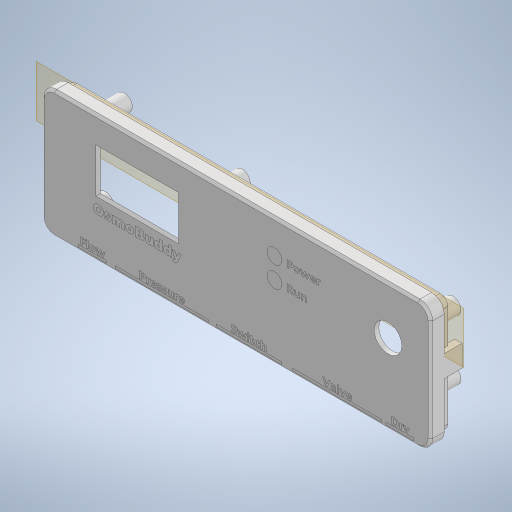
# Autodesk Inventor part: osmobuddy_top
Saved by Autodesk Inventor 2024.3 (Build 283343000, 343)
## iProperties
Created: 2024-10-17
Part Number: osmobuddy_top
Material: Generic
Document SubType Name: Modeling
Designer: atrus
Density: 1 g/cm^3
Appearance: Default
Author: atrus
Autodesk Inventor part; units mm, degrees
(part 1 of 2)
ref_plane "YZ Plane" through (0, 0, 0) normal (1, 0, 0) x (0, 1, 0)
ref_plane "XZ Plane" through (0, 0, 0) normal (0, 1, 0) x (-1, 0, 0)
ref_plane "Work Plane1" through (0, 0, 0) normal (0, 0, 1) x (1, 0, 0)
sketch "Sketch1" plane through (0, 0, 0) normal (0, 0, 1) x (1, 0, 0)
  line L0 (-78.5, 27.45) -> (78.5, 27.45)
  arc A0 (-78.5, 27.45) -> (-83.95, 22) centre (-78.5, 22) ccw
  line L1 (-83.95, -22) -> (-83.95, -15.775)
  arc A1 (-83.95, -22) -> (-78.5, -27.45) centre (-78.5, -22) ccw
  arc A2 (78.5, -27.45) -> (83.95, -22) centre (78.5, -22) ccw
  line L2 (83.95, -3.086) -> (83.95, -22)
  arc A3 (83.95, 22) -> (78.5, 27.45) centre (78.5, 22) ccw
  line L3 (83.95, 22) -> (83.95, -3.086)
  line L4 (-83.95, 22) -> (-83.95, -15.775)
  line L5 (-78.5, -27.45) -> (78.5, -27.45)
  point P0 (0, 0)
extrude "Extrusion1" add sketch "Sketch1" along normal blind 6
sketch "Sketch2" plane through (0, 0, 0) normal (0, 0, -1) x (-1, 0, 0)
  arc A0 (-78.5, 25.5) -> (-82, 22) centre (-78.5, 22) ccw projected
  line L0 (-78.5, 25.5) -> (61.235, 25.5) projected
  arc A1 (82, 22) -> (78.5, 25.5) centre (78.5, 22) ccw projected
  arc A2 (78.5, -25.5) -> (82, -22) centre (78.5, -22) ccw projected
  arc A3 (-82, -22) -> (-78.5, -25.5) centre (-78.5, -22) ccw projected
  line L1 (-82, 22) -> (-82, -22)
  line L2 (-78.5, 25.5) -> (78.5, 25.5)
  line L3 (82, 22) -> (82, -22)
  line L4 (83.95, 22) -> (83.95, -22) projected
  line L5 (78.5, -25.5) -> (-78.5, -25.5)
  line L6 (78.5, -27.45) -> (-78.5, -27.45) projected
  arc A4 (-78.5, 25.3) -> (-81.8, 22) centre (-78.5, 22) ccw
  line L7 (-78.5, 25.3) -> (78.5, 25.3)
  arc A5 (81.8, 22) -> (78.5, 25.3) centre (78.5, 22) ccw
  line L8 (81.8, 22) -> (81.8, -22)
  arc A6 (78.5, -25.3) -> (81.8, -22) centre (78.5, -22) ccw
  line L9 (78.5, -25.3) -> (-78.5, -25.3)
  arc A7 (-81.8, -22) -> (-78.5, -25.3) centre (-78.5, -22) ccw
  line L10 (-81.8, -22) -> (-81.8, 22)
  line L11 (78.5, 24.3) -> (-78.5, 24.3)
  arc A8 (-78.5, 24.3) -> (-80.8, 22) centre (-78.5, 22) ccw
  line L12 (-80.8, 22) -> (-80.8, -22)
  arc A9 (-80.8, -22) -> (-78.5, -24.3) centre (-78.5, -22) ccw
  line L13 (-78.5, -24.3) -> (78.5, -24.3)
  arc A10 (78.5, -24.3) -> (80.8, -22) centre (78.5, -22) ccw
  line L14 (80.8, -22) -> (80.8, 22)
  arc A11 (80.8, 22) -> (78.5, 24.3) centre (78.5, 22) ccw
  point P0 (0, 0)
  dimension "d2" = 0.2
  dimension "d3" = 1
  constraints: 24 end point, 16 point on circle, 8 centre point, 2 parallel, 1 collinear, 14 other
  measures "d2" distance between parallel lines of L0 L7
  measures "d3" distance between parallel lines of L7 L11
extrude "Extrusion2" add sketch "Sketch2" along normal blind 3.7 contours L7 A5 L8 A6 L9 A7 L10 A4
sketch "Sketch12" plane through (0, 0, 0) normal (0, 0, -1) x (-1, 0, 0)
  line L0 (78.5, 24.3) -> (-78.5, 24.3) projected
  arc A0 (-78.5, 24.3) -> (-80.8, 22) centre (-78.5, 22) ccw projected
  line L1 (-80.8, 22) -> (-80.8, -22) projected
  arc A1 (-80.8, -22) -> (-78.5, -24.3) centre (-78.5, -22) ccw projected
  line L2 (-78.5, -24.3) -> (78.5, -24.3) projected
  arc A2 (78.5, -24.3) -> (80.8, -22) centre (78.5, -22) ccw projected
  line L3 (80.8, -22) -> (80.8, 22) projected
  arc A3 (80.8, 22) -> (78.5, 24.3) centre (78.5, 22) ccw projected
  point P0 (0, 0)
extrude "Extrusion12" cut sketch "Sketch12" against normal blind 4
sketch "Sketch3" plane through (0, 0, 4) normal (0, 0, -1) x (-1, 0, 0)
  circle A0 centre (-76.5, 16) radius 1.8 construction
  circle A1 centre (-76.5, -10) radius 1.8 construction
  circle A2 centre (14.5, 18) radius 1.8 construction
  circle A3 centre (14.5, -8) radius 1.8 construction
  circle A4 centre (65.5, 21) radius 1.8 construction
  circle A5 centre (73.5, -20) radius 1.8 construction
  circle A6 centre (-76.5, 16) radius 3.5
  circle A7 centre (-76.5, -10) radius 3.5
  circle A8 centre (14.5, 18) radius 3.5
  circle A9 centre (14.5, -8) radius 3.5
  circle A10 centre (65.5, 21) radius 3.5
  circle A11 centre (73.5, -20) radius 3.5
  point P0 (0, 0)
  dimension "d6" = 7
  constraints: 6 centre point, 6 coincident, 5 equal radius
  measures "d6" diameter of A6
ref_plane "Work Plane2" through (-89.65, -27.5, -11.2032) normal (0, 0, 1) x (1, 0, 0)
extrude "Extrusion3" add sketch "Sketch3" along normal up to surface (15.2032 mm away)
sketch "Sketch4" plane through (0, 0, 6) normal (0, 0, 1) x (1, 0, 0)
  arc A0 (63.3499, 8.5) -> (67.9502, 8.5) centre (65.65, 7) ccw construction
  circle A1 centre (65.65, 7) radius 6
  line L0 (-59.595, 15.12) -> (-25.945, 15.12)
  line L1 (-25.945, 15.12) -> (-25.945, -2.08)
  line L2 (-25.945, -2.08) -> (-59.595, -2.08)
  line L3 (-59.595, -2.08) -> (-59.595, 15.12)
  line L4 (78.5, 27.45) -> (-78.5, 27.45) projected
  circle A2 centre (-44.04, 20) radius 0.508 projected
  circle A3 centre (-41.5, 20) radius 0.508 projected
  line L5 (-44.04, 20) -> (-41.5, 20) construction
  line L6 (-42.77, 20) -> (-42.77, -6.787) construction
  point P0 (0, 0)
  point P1 (-42.77, 15.12)
  dimension "d9" = 12
  dimension "d10" = 12.33
  dimension "d11" = 33.65
  dimension "d12" = 17.2
  constraints: 12 end point, 2 horizontal, 2 midpoint, 2 parallel, 1 centre point, 1 coincident, 1 perpendicular, 1 point on line, 1 vertical
  measures "d9" diameter of A1
  measures "d10" distance from line of L4 L0.end
  measures "d11" distance of L0.start L0.end
  measures "d12" distance of L0.end L1.end
extrude "Extrusion4" cut sketch "Sketch4" against normal blind 10 contours A1 | L0 L1 L2 L3
sketch "Sketch5" plane through (-83.95, -22, 0) normal (-1, 0, 0) x (0, 0, 1)
  line L0 (0, 39.12) -> (0, 20.92) projected
  line L1 (0, 33.7998) -> (-21.3034, 33.7998)
  line L2 (-21.3034, 33.7998) -> (-21.3034, 43.1998)
  line L3 (-21.3034, 43.1998) -> (0, 43.1998)
  line L4 (0, 43.1998) -> (0, 33.7998)
  line L5 (-11.4032, 43.1998) -> (0, 43.1998) construction
  line L6 (-11.2032, 33.9998) -> (-0.2032, 33.9998) construction
  line L7 (-0.2032, 33.9998) -> (-0.2032, 42.9998) projected
  line L8 (-0.2032, 38.4998) -> (5.1502, 38.4998) construction
  line L9 (-3.3332, 27.4) -> (-1.945, 27.4) construction
  line L10 (-1.945, 26.1) -> (-3.3332, 26.1) construction
  line L11 (-3.3332, 27.4) -> (-1.945, 27.4) construction
  line L12 (-1.945, 26.1) -> (-3.3332, 26.1) construction
  line L13 (0, 28.25) -> (-5.2744, 28.25)
  line L14 (-5.2744, 28.25) -> (-5.2744, 25.25)
  line L15 (-5.2744, 25.25) -> (0, 25.25)
  line L16 (0, 25.25) -> (0, 28.25)
  line L17 (-2.6391, 27.4) -> (-2.6391, 26.1) construction
  line L18 (-2.6391, 26.75) -> (7.1194, 26.75) construction
  line L19 (-3.3332, 13.65) -> (-1.945, 13.65) construction
  line L20 (-3.3332, 13.65) -> (-3.3332, 12.35) construction
  line L21 (-1.945, 12.35) -> (-3.3332, 12.35) construction
  line L22 (-1.945, 13.65) -> (-1.945, 12.35) construction
  line L23 (-1.945, 13) -> (5.1502, 13) construction
  line L24 (0, 0) -> (0, 44) projected
  line L25 (0, 14.5) -> (-4.6884, 14.5)
  line L26 (-4.6884, 14.5) -> (-4.6884, 11.5)
  line L27 (-4.6884, 11.5) -> (0, 11.5)
  line L28 (0, 11.5) -> (0, 14.5)
  point P0 (0, 22)
  point P1 (0, 38.4998)
  point P2 (0, 26.75)
  point P3 (-2.6372, 28.25)
  point P4 (0, 13)
  point P5 (-2.3442, 11.5)
  point P6 (-2.3442, 14.5)
  point P7 (0, 11.5)
  dimension "d15" = 3
  dimension "d16" = 3
  constraints: 32 end point, 11 midpoint, 6 horizontal, 6 parallel, 6 point on line, 3 perpendicular, 2 other
  measures "d15" distance from line of L15 point (-2.637, 28.25)
  measures "d16" distance of point (-2.344, 11.5) point (-2.344, 14.5)
extrude "Extrusion5" cut sketch "Sketch5" against normal blind 10
sketch "Sketch6" plane through (0, 0, 0) normal (0, 0, -1) x (-1, 0, 0)
  line L0 (-83.95, -22) -> (-83.95, 22) projected
  line L1 (-83.95, 7.254) -> (-80.8, 7.254)
  line L2 (-80.8, 7.254) -> (-80.8, -2.086)
  line L3 (-80.8, -2.086) -> (-83.95, -2.086)
  line L4 (-83.95, -2.086) -> (-83.95, 7.254)
  line L5 (-80.8, -22) -> (-80.8, 22) projected
  point P0 (0, 0)
  point P1 (-82.95, -2.086)
  point P2 (-82.95, 7.254)
  point P3 (-80.8, 2.584)
  constraints: 8 end point, 4 point on line, 2 parallel, 1 horizontal, 1 midpoint, 1 perpendicular, 2 other
extrude "Extrusion6" add sketch "Sketch6" along normal blind 7.7
sketch "Sketch7" plane through (0, 0, 0) normal (0, 0, -1) x (-1, 0, 0)
  line L0 (78.5, -27.45) -> (-78.5, -27.45) projected
  line L1 (78.5, -24.3) -> (-78.5, -24.3) projected
  line L2 (-65.1727, -27.45) -> (-76.779, -27.45)
  line L3 (-76.779, -27.45) -> (-76.779, -24.3)
  line L4 (-76.779, -24.3) -> (-65.1727, -24.3)
  line L5 (-65.1727, -24.3) -> (-65.1727, -27.45)
  line L6 (-62.93, -27.45) -> (-54.52, -27.45)
  line L7 (-54.52, -27.45) -> (-54.52, -24.3)
  line L8 (-54.52, -24.3) -> (-62.93, -24.3)
  line L9 (-62.93, -24.3) -> (-62.93, -27.45)
  line L10 (-52.5337, -27.45) -> (-44.52, -27.45)
  line L11 (-44.52, -27.45) -> (-44.52, -24.3)
  line L12 (-44.52, -24.3) -> (-52.5337, -24.3)
  line L13 (-52.5337, -24.3) -> (-52.5337, -27.45)
  line L14 (-42.93, -27.45) -> (-34.52, -27.45)
  line L15 (-34.52, -27.45) -> (-34.52, -24.3)
  line L16 (-34.52, -24.3) -> (-42.93, -24.3)
  line L17 (-42.93, -24.3) -> (-42.93, -27.45)
  line L18 (-32.93, -27.45) -> (-24.52, -27.45)
  line L19 (-24.52, -27.45) -> (-24.52, -24.3)
  line L20 (-24.52, -24.3) -> (-32.93, -24.3)
  line L21 (-32.93, -24.3) -> (-32.93, -27.45)
  line L22 (-24.12, -27.45) -> (-20.14, -27.45)
  line L23 (-20.14, -27.45) -> (-20.14, -24.3)
  line L24 (-20.14, -24.3) -> (-24.12, -24.3)
  line L25 (-24.12, -24.3) -> (-24.12, -27.45)
  line L26 (-19.6962, -27.45) -> (-11.33, -27.45)
  line L27 (-11.33, -27.45) -> (-11.33, -24.3)
  line L28 (-11.33, -24.3) -> (-19.6962, -24.3)
  line L29 (-19.6962, -24.3) -> (-19.6962, -27.45)
  line L30 (-9.74, -27.45) -> (-1.33, -27.45)
  line L31 (-1.33, -27.45) -> (-1.33, -24.3)
  line L32 (-1.33, -24.3) -> (-9.74, -24.3)
  line L33 (-9.74, -24.3) -> (-9.74, -27.45)
  line L34 (8.67, -24.3) -> (0, -24.3)
  line L35 (12.221, -27.45) -> (24.241, -27.45)
  line L36 (24.241, -27.45) -> (24.241, -24.3)
  line L37 (24.241, -24.3) -> (12.221, -24.3)
  line L38 (12.221, -24.3) -> (12.221, -27.45)
  line L39 (26.221, -27.45) -> (38.241, -27.45)
  line L40 (38.241, -27.45) -> (38.241, -24.3)
  line L41 (38.241, -24.3) -> (26.221, -24.3)
  line L42 (26.221, -24.3) -> (26.221, -27.45)
  line L43 (40.221, -27.45) -> (52.241, -27.45)
  line L44 (52.241, -27.45) -> (52.241, -24.3)
  line L45 (52.241, -24.3) -> (40.221, -24.3)
  line L46 (40.221, -24.3) -> (40.221, -27.45)
  line L47 (56.021, -27.45) -> (68.241, -27.45)
  line L48 (68.241, -27.45) -> (68.241, -24.3)
  line L49 (68.241, -24.3) -> (56.021, -24.3)
  line L50 (56.021, -24.3) -> (56.021, -27.45)
  line L51 (0.2, -27.45) -> (8.67, -27.45)
  line L52 (8.67, -27.45) -> (8.67, -24.3)
  line L53 (8.67, -24.3) -> (0.2, -24.3)
  line L54 (0.2, -24.3) -> (0.2, -27.45)
  point P0 (0, 0)
  point P1 (68.441, -27.45)
  point P2 (55.821, -27.45)
  point P3 (52.441, -27.45)
  point P4 (40.021, -35.16)
  point P5 (38.441, -27.45)
  point P6 (26.021, -35.16)
  point P7 (24.441, -27.45)
  point P8 (12.021, -35.16)
  point P9 (8.87, -27.45)
  point P10 (0, -27.45)
  point P11 (-1.13, -27.45)
  point P12 (-9.94, -27.45)
  point P13 (-11.13, -27.45)
  point P14 (-19.94, -27.45)
  point P15 (-24.32, -27.45)
  point P16 (-33.13, -27.45)
  point P17 (-34.32, -27.45)
  point P18 (-43.13, -27.45)
  point P19 (-44.32, -27.45)
  point P20 (-53.13, -27.45)
  point P21 (-54.32, -27.45)
  point P22 (-63.13, -27.45)
  point P23 (-64.559, -27.45)
  point P24 (-76.979, -35.16)
  point P25 (52.241, -25.875)
  point P26 (56.021, -25.875)
  point P27 (24.241, -25.875)
  point P28 (12.221, -25.875)
  point P29 (0, -27.45)
  point P30 (-19.6962, -25.875)
  point P31 (-20.14, -25.875)
  point P32 (-24.12, -25.875)
  point P33 (56.021, -24.3)
  point P34 (68.241, -24.3)
  point P35 (40.221, -24.3)
  point P36 (52.241, -24.3)
  point P37 (26.221, -24.3)
  point P38 (38.241, -24.3)
  point P39 (12.221, -24.3)
  point P40 (24.241, -24.3)
  point P41 (0.2, -24.3)
  point P42 (8.67, -24.3)
  point P43 (-9.74, -24.3)
  point P44 (-1.33, -27.45)
  point P45 (-1.33, -24.3)
  point P46 (-19.6962, -24.3)
  point P47 (-11.33, -24.3)
  point P48 (-32.93, -24.3)
  point P49 (-24.52, -24.3)
  point P50 (-42.93, -24.3)
  point P51 (-34.52, -27.45)
  point P52 (-34.52, -24.3)
  point P53 (-52.5337, -24.3)
  point P54 (-44.52, -24.3)
  point P55 (-62.93, -24.3)
  point P56 (-54.52, -24.3)
  point P57 (-65.1727, -24.3)
  point P58 (-76.779, -27.45)
  dimension "d21" = 0.2
  dimension "d22" = 0.2
  dimension "d23" = 0.2
  dimension "d24" = 0.2
  dimension "d25" = 0.2
  dimension "d26" = 0.2
  dimension "d27" = 0.2
  dimension "d28" = 0.2
  dimension "d30" = 0.2
  dimension "d31" = 0.2
  dimension "d32" = 0.2
  dimension "d33" = 0.2
  dimension "d34" = 0.2
  dimension "d35" = 1.575
  dimension "d36" = 0.2
  dimension "d37" = 0.2
  dimension "d38" = 0.2
  dimension "d39" = 0.2
  dimension "d40" = 0.2
  dimension "d41" = 0.2
  dimension "d42" = 0.2
  dimension "d43" = 0.2
  dimension "d44" = 0.2
  dimension "d45" = 0.2
  constraints: 106 end point, 26 parallel, 23 point on line, 13 horizontal, 13 perpendicular, 7 midpoint, 30 other
  measures "d21" distance from line of L46 point (40.021, -35.16)
  measures "d22" horizontal distance of point (52.241, -25.875) point (52.441, -27.45)
  measures "d23" horizontal distance of point (56.021, -25.875) point (55.821, -27.45)
  measures "d24" distance from line of point (68.441, -27.45) L48
  measures "d25" distance from line of point (38.441, -27.45) L40
  measures "d26" distance from line of L42 point (26.021, -35.16)
  measures "d27" horizontal distance of point (24.241, -25.875) point (24.441, -27.45)
  measures "d28" horizontal distance of point (12.021, -35.16) point (12.221, -25.875)
  measures "d30" distance from line of L54 point (0, -27.45)
  measures "d31" distance from line of L52 point (8.87, -27.45)
  measures "d32" distance from line of point (-1.13, -27.45) L31
  measures "d33" distance from line of L33 point (-9.94, -27.45)
  measures "d34" distance from line of point (-11.13, -27.45) L27
  measures "d35" vertical distance of point (-19.696, -25.875) point (-19.94, -27.45)
  measures "d36" horizontal distance of point (-20.14, -25.875) point (-19.94, -27.45)
  measures "d37" horizontal distance of point (-24.12, -25.875) point (-24.32, -27.45)
  measures "d38" distance from line of point (-24.32, -27.45) L19
  measures "d39" distance from line of L21 point (-33.13, -27.45)
  measures "d40" distance from line of point (-34.32, -27.45) L15
  measures "d41" distance from line of L3 point (-76.979, -35.16)
  measures "d42" distance from line of L9 point (-63.13, -27.45)
  measures "d43" distance from line of L7 point (-54.32, -27.45)
  measures "d44" distance from line of point (-44.32, -27.45) L11
  measures "d45" distance from line of point (-43.13, -27.45) L17
extrude "Extrusion7" add sketch "Sketch7" along normal blind 3.7 contours L0 L50 L1 L48 | L0 L46 L1 L44 | L0 L42 L1 L40 | L0 L38 L1 L36 | L0 L54 L1 L52 | L0 L33 L1 L31 | L0 L29 L1 L27 | L0 L21 L1 L19 | L0 L17 L1 L15 | L0 L13 L1 L11 | L0 L9 L1 L7 | L0 L3 L1 L5
sketch "Sketch8" plane through (76.5, 16, -11.2032) normal (0, 0, -1) x (-1, 0, 0)
  circle A0 centre (0, 0) radius 3.5 construction
  circle A1 centre (0, -26) radius 3.5 construction
  circle A2 centre (91, -24) radius 3.5 construction
  circle A3 centre (91, 2) radius 3.5 construction
  circle A4 centre (142, 5) radius 3.5 construction
  circle A5 centre (150, -36) radius 3.5 construction
  circle A6 centre (0, 0) radius 2
  circle A7 centre (0, -26) radius 2
  circle A8 centre (91, 2) radius 2
  circle A9 centre (91, -24) radius 2
  circle A10 centre (142, 5) radius 2
  circle A11 centre (150, -36) radius 2
  point P0 (76.5, -16)
  dimension "d48" = 4
  constraints: 6 centre point, 6 coincident, 5 equal radius
  measures "d48" diameter of A6
extrude "Extrusion8" cut sketch "Sketch8" against normal blind 7
chamfer "Chamfer1" distance 1 angle 45 12 edges at (-42.77, 15.12, 6) (-25.945, 6.52, 6) (-42.77, -2.08, 6) (-59.595, 6.52, 6) (-83.95, 0, 6) (-82.3537, -25.8537, 6) (0, -27.45, 6) (82.3537, -25.8537, 6) (83.95, 0, 6) (82.3537, 25.8537, 6) (0, 27.45, 6) (-82.3537, 25.8537, 6)
sketch "Sketch9" plane through (0, 0, 4) normal (0, 0, -1) x (-1, 0, 0)
  arc A0 (-19.1701, 11.4418) -> (-19.1701, 14.7584) centre (-16.6701, 13.1001) ccw projected
  arc A1 (-19.1701, 2.4418) -> (-19.1701, 5.7584) centre (-16.6701, 4.1001) ccw projected
  circle A2 centre (-16.6701, 13.1001) radius 3.2
  circle A3 centre (-16.6701, 4.1001) radius 3.2
  circle A4 centre (-16.6701, 13.1001) radius 4.2
  circle A5 centre (-16.6701, 4.1001) radius 4.2
  point P0 (0, 0)
  dimension "d54" = 0.2
  dimension "d55" = 1
  constraints: 4 centre point, 2 coincident, 2 equal radius
  measures "d54" radial gap between concentric circles of A2 A0
  measures "d55" radial gap between concentric circles of A4 A2
extrude "Extrusion9" add sketch "Sketch9" along normal blind 10
sketch "Sketch10" plane through (16.6701, 13.1001, 0) normal (0, 0, -1) x (-1, 0, 0)
  circle A0 centre (0, 0) radius 3.2 projected
  circle A1 centre (0, -9) radius 3.2 projected
  point P0 (16.6701, -13.1001)
extrude "Extrusion10" cut sketch "Sketch10" against normal blind 5.6
sketch "Sketch11" plane through (0, 0, 6) normal (0, 0, 1) x (1, 0, 0)
  line L0 (-24.945, -3.08) -> (-24.945, 16.12) projected
  line L1 (-60.595, -3.08) -> (-24.945, -3.08) projected
  line L2 (-60.595, 16.12) -> (-60.595, -3.08) projected
  line L3 (-24.945, 16.12) -> (-60.595, 16.12) projected
  circle A0 centre (65.65, 7) radius 6 projected
  line L4 (-82.95, -22) -> (-82.95, 22) projected
  arc A1 (-82.95, -22) -> (-78.5, -26.45) centre (-78.5, -22) ccw projected
  line L5 (78.5, -26.45) -> (-78.5, -26.45) projected
  arc A2 (78.5, -26.45) -> (82.95, -22) centre (78.5, -22) ccw projected
  line L6 (82.95, 22) -> (82.95, -22) projected
  arc A3 (82.95, 22) -> (78.5, 26.45) centre (78.5, 22) ccw projected
  line L7 (-78.5, 26.45) -> (78.5, 26.45) projected
  arc A4 (-78.5, 26.45) -> (-82.95, 22) centre (-78.5, 22) ccw projected
  circle A5 centre (16.6701, 13.1001) radius 3.2 projected
  circle A6 centre (16.6701, 4.1001) radius 3.2 projected
  point P0 (0, 0)
extrude "Extrusion11" cut sketch "Sketch11" against normal blind 0.001 contours A5 | A6
sketch "Sketch13" plane through (0, 0, 4) normal (0, 0, -1) x (-1, 0, 0)
  line L0 (23.945, 21.12) -> (61.595, 21.12)
  line L1 (61.595, 21.12) -> (61.595, -8.08)
  line L2 (61.595, -8.08) -> (23.945, -8.08)
  line L3 (23.945, -8.08) -> (23.945, 21.12)
  line L4 (59.595, -2.08) -> (25.945, -2.08) projected
  line L5 (25.945, -2.08) -> (25.945, 15.12) projected
  line L6 (59.595, 15.12) -> (59.595, -2.08) projected
  line L7 (25.945, 15.12) -> (59.595, 15.12) projected
  point P0 (0, 0)
  point P1 (42.77, -2.08)
  point P2 (42.77, -8.08)
  point P3 (42.77, 15.12)
  dimension "d64" = 6
  dimension "d65" = 2
  dimension "d66" = 2
  dimension "d67" = 6
  constraints: 8 end point, 3 midpoint, 2 parallel, 1 horizontal, 1 perpendicular
  measures "d64" distance of point (42.77, -2.08) point (42.77, -8.08)
  measures "d65" distance between parallel lines of L5 L3
  measures "d66" distance between parallel lines of L6 L1
  measures "d67" distance from line of point (42.77, 15.12) L0
extrude "Extrusion13" cut sketch "Sketch13" against normal blind 1
sketch "Sketch14" plane through (0, 0, 6) normal (0, 0, 1) x (1, 0, 0)
  line L0 (-68.241, -24.56) -> (-56.021, -24.56) construction
  line L1 (-68.241, -28.56) -> (-68.241, -35.16) construction
  line L2 (-56.021, -28.56) -> (-56.021, -35.16) construction
  line L3 (-52.241, -28.56) -> (-52.241, -35.16) construction
  line L4 (-12.021, -28.56) -> (-12.021, -35.16) construction
  line L5 (-8.67, -34.606) -> (-8.67, -28.806) construction
  line L6 (19.74, -34.606) -> (19.74, -28.806) construction
  line L7 (-52.241, -24.56) -> (-12.021, -24.56) construction
  line L8 (-8.67, -24.56) -> (19.74, -24.56) construction
  line L9 (62.93, -34.606) -> (62.93, -28.806) construction
  line L10 (64.759, -28.56) -> (64.759, -35.16) construction
  line L11 (76.979, -28.56) -> (76.979, -35.16) construction
  line L12 (24.52, -24.56) -> (62.93, -24.56) construction
  line L13 (24.52, -34.606) -> (24.52, -28.806) construction
  line L14 (64.759, -28.56) -> (64.759, -35.16) construction
  line L15 (76.979, -28.56) -> (76.979, -35.16) construction
  line L16 (64.759, -24.56) -> (76.979, -24.56) construction
  line L17 (-52.241, -24.96) -> (-12.021, -24.96)
  line L18 (-12.021, -24.96) -> (-12.021, -25.96)
  line L19 (-12.021, -25.96) -> (-52.241, -25.96)
  line L20 (-52.241, -25.96) -> (-52.241, -24.96)
  line L21 (-68.241, -25.3) -> (-68.241, -27.45) projected
  line L22 (-56.021, -24.96) -> (-68.241, -24.96)
  line L23 (-68.241, -24.96) -> (-68.241, -25.96)
  line L24 (-68.241, -25.96) -> (-56.021, -25.96)
  line L25 (-56.021, -25.96) -> (-56.021, -24.96)
  line L26 (-8.67, -25.3) -> (-8.67, -27.45) projected
  line L27 (-8.67, -25.96) -> (19.74, -25.96)
  line L28 (19.74, -25.96) -> (19.74, -24.96)
  line L29 (19.74, -24.96) -> (-8.67, -24.96)
  line L30 (-8.67, -24.96) -> (-8.67, -25.96)
  line L31 (24.52, -25.96) -> (62.93, -25.96)
  line L32 (62.93, -25.96) -> (62.93, -24.96)
  line L33 (62.93, -24.96) -> (24.52, -24.96)
  line L34 (24.52, -24.96) -> (24.52, -25.96)
  line L35 (76.779, -25.3) -> (76.779, -27.45) projected
  line L36 (64.759, -24.96) -> (76.779, -24.96)
  line L37 (76.779, -24.96) -> (76.779, -25.96)
  line L38 (76.779, -25.96) -> (64.759, -25.96)
  line L39 (64.759, -25.96) -> (64.759, -24.96)
  circle A0 centre (16.6701, 13.1001) radius 3.2 construction
  circle A1 centre (16.6701, 4.1001) radius 3.2 construction
  line L40 (16.6701, 13.1001) -> (16.6701, 9.9001) construction
  line L41 (16.6701, 4.1001) -> (16.6701, 0.9001) construction
  line L42 (16.6701, 2.5001) -> (21.6701, 2.5001) construction
  line L43 (16.6701, 11.5001) -> (21.6701, 11.5001) construction
  line L44 (-61.8904, -9.6935) -> (-23.2153, -9.6935) construction
  line L45 (-64.9786, -22.076) -> (-64.9786, -21.51)
  line L46 (-64.9786, -21.51) -> (-67.2837, -21.51)
  line L47 (-67.2837, -21.51) -> (-67.2837, -24.56)
  line L48 (-67.2837, -24.56) -> (-66.577, -24.56)
  line L49 (-66.577, -24.56) -> (-66.577, -23.4485)
  line L50 (-66.577, -23.4485) -> (-65.1663, -23.4485)
  line L51 (-65.1663, -23.4485) -> (-65.1663, -22.8825)
  line L52 (-65.1663, -22.8825) -> (-66.577, -22.8825)
  line L53 (-66.577, -22.8825) -> (-66.577, -22.076)
  line L54 (-66.577, -22.076) -> (-64.9786, -22.076)
  line L55 (-64.5475, -24.56) -> (-63.8672, -24.56)
  line L56 (-63.8672, -24.56) -> (-63.8672, -21.3282)
  line L57 (-63.8672, -21.3282) -> (-64.5475, -21.3282)
  line L58 (-64.5475, -21.3282) -> (-64.5475, -24.56)
  spline S0 degree 2 poles (-62.1222, -24.5952) (-61.7468, -24.5923) (-61.1691, -24.2873) (-60.8406, -23.7447) (-60.8377, -23.3869) knots 0 0 0 1 2 3 3 3
  spline S1 degree 2 poles (-60.8377, -23.3869) (-60.8406, -23.0321) (-61.1691, -22.4895) (-61.7468, -22.1845) (-62.1222, -22.1816) knots 0 0 0 1 2 3 3 3
  spline S2 degree 2 poles (-62.1222, -22.1816) (-62.4976, -22.1845) (-63.0783, -22.4895) (-63.4097, -23.0321) (-63.4126, -23.3869) knots 0 0 0 1 2 3 3 3
  spline S3 degree 2 poles (-63.4126, -23.3869) (-63.4097, -23.7447) (-63.0783, -24.2873) (-62.4976, -24.5923) (-62.1222, -24.5952) knots 0 0 0 1 2 3 3 3
  spline S4 degree 2 poles (-62.1222, -24.038) (-62.3832, -24.035) (-62.7175, -23.6949) (-62.7234, -23.3869) knots 0 0 0 1 2 2 2
  spline S5 degree 2 poles (-62.7234, -23.3869) (-62.7175, -23.0819) (-62.3832, -22.7417) (-62.1222, -22.7388) knots 0 0 0 1 2 2 2
  spline S6 degree 2 poles (-62.1222, -22.7388) (-61.8641, -22.7417) (-61.5327, -23.0819) (-61.5269, -23.3869) knots 0 0 0 1 2 2 2
  spline S7 degree 2 poles (-61.5269, -23.3869) (-61.5327, -23.6949) (-61.8641, -24.035) (-62.1222, -24.038) knots 0 0 0 1 2 2 2
  line L59 (-57.2217, -22.2168) -> (-57.7935, -23.8034)
  line L60 (-57.7935, -23.8034) -> (-58.3508, -22.2168)
  line L61 (-58.3508, -22.2168) -> (-58.9256, -22.2168)
  line L62 (-58.9256, -22.2168) -> (-59.5004, -23.8034)
  line L63 (-59.5004, -23.8034) -> (-60.0547, -22.2168)
  line L64 (-60.0547, -22.2168) -> (-60.694, -22.2168)
  line L65 (-60.694, -22.2168) -> (-59.8494, -24.56)
  line L66 (-59.8494, -24.56) -> (-59.1954, -24.56)
  line L67 (-59.1954, -24.56) -> (-58.6499, -23.1054)
  line L68 (-58.6499, -23.1054) -> (-58.1249, -24.56)
  line L69 (-58.1249, -24.56) -> (-57.471, -24.56)
  line L70 (-57.471, -24.56) -> (-56.6205, -22.2168)
  line L71 (-56.6205, -22.2168) -> (-57.2217, -22.2168)
  line L72 (-40.4789, -21.51) -> (-41.7986, -21.51)
  line L73 (-41.7986, -21.51) -> (-41.7986, -24.56)
  line L74 (-41.7986, -24.56) -> (-41.0918, -24.56)
  line L75 (-41.0918, -24.56) -> (-41.0918, -23.7183)
  line L76 (-41.0918, -23.7183) -> (-40.4789, -23.7183)
  spline S8 degree 2 poles (-40.4789, -23.7183) (-39.8601, -23.7125) (-39.1592, -23.1318) (-39.1533, -22.6156) knots 0 0 0 1 2 2 2
  spline S9 degree 2 poles (-39.1533, -22.6156) (-39.1592, -22.0995) (-39.8601, -21.5159) (-40.4789, -21.51) knots 0 0 0 1 2 2 2
  line L77 (-40.517, -23.1435) -> (-41.0918, -23.1435)
  line L78 (-41.0918, -23.1435) -> (-41.0918, -22.0848)
  line L79 (-41.0918, -22.0848) -> (-40.517, -22.0848)
  spline S10 degree 2 poles (-40.517, -22.0848) (-40.1944, -22.0877) (-39.8689, -22.3634) (-39.8689, -22.6156) knots 0 0 0 1 2 2 2
  spline S11 degree 2 poles (-39.8689, -22.6156) (-39.8689, -22.8678) (-40.1944, -23.1406) (-40.517, -23.1435) knots 0 0 0 1 2 2 2
  line L80 (-38.0096, -22.5247) -> (-38.0096, -22.2168)
  line L81 (-38.0096, -22.2168) -> (-38.6577, -22.2168)
  line L82 (-38.6577, -22.2168) -> (-38.6577, -24.56)
  line L83 (-38.6577, -24.56) -> (-37.9773, -24.56)
  line L84 (-37.9773, -24.56) -> (-37.9773, -23.4544)
  spline S12 degree 2 poles (-37.9773, -23.4544) (-37.9744, -23.1171) (-37.6401, -22.8004) (-37.3556, -22.8004) knots 0 0 0 1 2 2 2
  spline S13 degree 2 poles (-37.3556, -22.8004) (-37.3175, -22.8004) (-37.2442, -22.8063) (-37.2031, -22.8092) knots 0 0 0 1 2 2 2
  line L85 (-37.2031, -22.8092) -> (-37.2031, -22.1816)
  spline S14 degree 2 poles (-37.2031, -22.1816) (-37.4758, -22.1816) (-37.8835, -22.3546) (-38.0096, -22.5247) knots 0 0 0 1 2 2 2
  spline S15 degree 2 poles (-34.4845, -23.3987) (-34.4874, -23.0174) (-34.8071, -22.4749) (-35.3555, -22.1845) (-35.7045, -22.1816) knots 0 0 0 1 2 3 3 3
  spline S16 degree 2 poles (-35.7045, -22.1816) (-36.0652, -22.1845) (-36.6254, -22.4925) (-36.9509, -23.035) (-36.9538, -23.3899) knots 0 0 0 1 2 3 3 3
  spline S17 degree 2 poles (-36.9538, -23.3899) (-36.9509, -23.7388) (-36.6224, -24.2814) (-36.0242, -24.5923) (-35.6165, -24.5952) knots 0 0 0 1 2 3 3 3
  spline S18 degree 2 poles (-35.6165, -24.5952) (-35.2998, -24.5952) (-34.8129, -24.4016) (-34.6487, -24.2169) knots 0 0 0 1 2 2 2
  line L86 (-34.6487, -24.2169) -> (-35.0124, -23.8239)
  spline S19 degree 2 poles (-35.0124, -23.8239) (-35.1297, -23.9383) (-35.4142, -24.0497) (-35.5989, -24.0497) knots 0 0 0 1 2 2 2
  spline S20 degree 2 poles (-35.5989, -24.0497) (-35.8687, -24.0468) (-36.2177, -23.8004) (-36.2705, -23.5805) knots 0 0 0 1 2 2 2
  line L87 (-36.2705, -23.5805) -> (-34.4992, -23.5805)
  spline S21 degree 2 poles (-34.4992, -23.5805) (-34.4933, -23.5365) (-34.4845, -23.4368) (-34.4845, -23.3987) knots 0 0 0 1 2 2 2
  spline S22 degree 2 poles (-35.6986, -22.6948) (-35.4669, -22.6977) (-35.1649, -22.9588) (-35.1238, -23.1846) knots 0 0 0 1 2 2 2
  line L88 (-35.1238, -23.1846) -> (-36.2793, -23.1846)
  spline S23 degree 2 poles (-36.2793, -23.1846) (-36.2412, -22.9558) (-35.9332, -22.6977) (-35.6986, -22.6948) knots 0 0 0 1 2 2 2
  spline S24 degree 2 poles (-33.244, -24.5952) (-32.7161, -24.5893) (-32.1413, -24.1846) (-32.1383, -23.8503) knots 0 0 0 1 2 2 2
  spline S25 degree 2 poles (-32.1383, -23.8503) (-32.1442, -23.5775) (-32.4287, -23.296) (-32.848, -23.1787) (-33.2674, -23.123) (-33.549, -23.0291) (-33.5548, -22.9148) knots 0 0 0 1 2 3 4 5 5 5
  spline S26 degree 2 poles (-33.5548, -22.9148) (-33.5578, -22.8209) (-33.3466, -22.6977) (-33.1179, -22.6948) knots 0 0 0 1 2 2 2
  spline S27 degree 2 poles (-33.1179, -22.6948) (-32.9566, -22.6919) (-32.6164, -22.774) (-32.4433, -22.8708) knots 0 0 0 1 2 2 2
  line L89 (-32.4433, -22.8708) -> (-32.2175, -22.3869)
  spline S28 degree 2 poles (-32.2175, -22.3869) (-32.3876, -22.2872) (-32.8715, -22.1816) (-33.1179, -22.1816) knots 0 0 0 1 2 2 2
  spline S29 degree 2 poles (-33.1179, -22.1816) (-33.634, -22.1875) (-34.2, -22.601) (-34.2029, -22.9412) knots 0 0 0 1 2 2 2
  spline S30 degree 2 poles (-34.2029, -22.9412) (-34.1971, -23.2168) (-33.9126, -23.5013) (-33.4932, -23.6215) (-33.0739, -23.6714) (-32.7923, -23.7594) (-32.7865, -23.8679) knots 0 0 0 1 2 3 4 5 5 5
  spline S31 degree 2 poles (-32.7865, -23.8679) (-32.7835, -23.9676) (-32.9859, -24.082) (-33.2176, -24.082) knots 0 0 0 1 2 2 2
  spline S32 degree 2 poles (-33.2176, -24.082) (-33.4404, -24.082) (-33.8716, -23.9588) (-34.0329, -23.8562) knots 0 0 0 1 2 2 2
  line L90 (-34.0329, -23.8562) -> (-34.2587, -24.343)
  spline S33 degree 2 poles (-34.2587, -24.343) (-34.0915, -24.4515) (-33.549, -24.5923) (-33.244, -24.5952) knots 0 0 0 1 2 2 2
  spline S34 degree 2 poles (-30.9301, -24.5952) (-30.4022, -24.5893) (-29.8274, -24.1846) (-29.8244, -23.8503) knots 0 0 0 1 2 2 2
  spline S35 degree 2 poles (-29.8244, -23.8503) (-29.8303, -23.5775) (-30.1148, -23.296) (-30.5342, -23.1787) (-30.9535, -23.123) (-31.2351, -23.0291) (-31.2409, -22.9148) knots 0 0 0 1 2 3 4 5 5 5
  spline S36 degree 2 poles (-31.2409, -22.9148) (-31.2439, -22.8209) (-31.0327, -22.6977) (-30.804, -22.6948) knots 0 0 0 1 2 2 2
  spline S37 degree 2 poles (-30.804, -22.6948) (-30.6427, -22.6919) (-30.3025, -22.774) (-30.1294, -22.8708) knots 0 0 0 1 2 2 2
  line L91 (-30.1294, -22.8708) -> (-29.9036, -22.3869)
  spline S38 degree 2 poles (-29.9036, -22.3869) (-30.0737, -22.2872) (-30.5576, -22.1816) (-30.804, -22.1816) knots 0 0 0 1 2 2 2
  spline S39 degree 2 poles (-30.804, -22.1816) (-31.3201, -22.1875) (-31.8861, -22.601) (-31.8891, -22.9412) knots 0 0 0 1 2 2 2
  spline S40 degree 2 poles (-31.8891, -22.9412) (-31.8832, -23.2168) (-31.5987, -23.5013) (-31.1793, -23.6215) (-30.76, -23.6714) (-30.4784, -23.7594) (-30.4726, -23.8679) knots 0 0 0 1 2 3 4 5 5 5
  spline S41 degree 2 poles (-30.4726, -23.8679) (-30.4696, -23.9676) (-30.672, -24.082) (-30.9037, -24.082) knots 0 0 0 1 2 2 2
  spline S42 degree 2 poles (-30.9037, -24.082) (-31.1266, -24.082) (-31.5577, -23.9588) (-31.719, -23.8562) knots 0 0 0 1 2 2 2
  line L92 (-31.719, -23.8562) -> (-31.9448, -24.343)
  spline S43 degree 2 poles (-31.9448, -24.343) (-31.7776, -24.4515) (-31.2351, -24.5923) (-30.9301, -24.5952) knots 0 0 0 1 2 2 2
  line L93 (-27.7246, -22.2168) -> (-27.7246, -23.3781)
  spline S44 degree 2 poles (-27.7246, -23.3781) (-27.7276, -23.7007) (-28.0238, -24.0087) (-28.2642, -24.0087) knots 0 0 0 1 2 2 2
  spline S45 degree 2 poles (-28.2642, -24.0087) (-28.493, -24.0116) (-28.7393, -23.7359) (-28.7393, -23.4426) knots 0 0 0 1 2 2 2
  line L94 (-28.7393, -23.4426) -> (-28.7393, -22.2168)
  line L95 (-28.7393, -22.2168) -> (-29.4197, -22.2168)
  line L96 (-29.4197, -22.2168) -> (-29.4197, -23.5424)
  spline S46 degree 2 poles (-29.4197, -23.5424) (-29.4168, -23.9031) (-29.1646, -24.3694) (-28.7129, -24.5952) (-28.4167, -24.5952) knots 0 0 0 1 2 3 3 3
  spline S47 degree 2 poles (-28.4167, -24.5952) (-28.1997, -24.5952) (-27.8243, -24.4368) (-27.6894, -24.2814) knots 0 0 0 1 2 2 2
  line L97 (-27.6894, -24.2814) -> (-27.6894, -24.56)
  line L98 (-27.6894, -24.56) -> (-27.0442, -24.56)
  line L99 (-27.0442, -24.56) -> (-27.0442, -22.2168)
  line L100 (-27.0442, -22.2168) -> (-27.7246, -22.2168)
  line L101 (-25.7656, -22.5247) -> (-25.7656, -22.2168)
  line L102 (-25.7656, -22.2168) -> (-26.4137, -22.2168)
  line L103 (-26.4137, -22.2168) -> (-26.4137, -24.56)
  line L104 (-26.4137, -24.56) -> (-25.7333, -24.56)
  line L105 (-25.7333, -24.56) -> (-25.7333, -23.4544)
  spline S48 degree 2 poles (-25.7333, -23.4544) (-25.7304, -23.1171) (-25.3961, -22.8004) (-25.1116, -22.8004) knots 0 0 0 1 2 2 2
  spline S49 degree 2 poles (-25.1116, -22.8004) (-25.0735, -22.8004) (-25.0002, -22.8063) (-24.9591, -22.8092) knots 0 0 0 1 2 2 2
  line L106 (-24.9591, -22.8092) -> (-24.9591, -22.1816)
  spline S50 degree 2 poles (-24.9591, -22.1816) (-25.2318, -22.1816) (-25.6395, -22.3546) (-25.7656, -22.5247) knots 0 0 0 1 2 2 2
  spline S51 degree 2 poles (-22.2405, -23.3987) (-22.2434, -23.0174) (-22.5631, -22.4749) (-23.1115, -22.1845) (-23.4605, -22.1816) knots 0 0 0 1 2 3 3 3
  spline S52 degree 2 poles (-23.4605, -22.1816) (-23.8212, -22.1845) (-24.3814, -22.4925) (-24.7069, -23.035) (-24.7098, -23.3899) knots 0 0 0 1 2 3 3 3
  spline S53 degree 2 poles (-24.7098, -23.3899) (-24.7069, -23.7388) (-24.3784, -24.2814) (-23.7802, -24.5923) (-23.3725, -24.5952) knots 0 0 0 1 2 3 3 3
  spline S54 degree 2 poles (-23.3725, -24.5952) (-23.0558, -24.5952) (-22.569, -24.4016) (-22.4047, -24.2169) knots 0 0 0 1 2 2 2
  line L107 (-22.4047, -24.2169) -> (-22.7684, -23.8239)
  spline S55 degree 2 poles (-22.7684, -23.8239) (-22.8857, -23.9383) (-23.1702, -24.0497) (-23.3549, -24.0497) knots 0 0 0 1 2 2 2
  spline S56 degree 2 poles (-23.3549, -24.0497) (-23.6247, -24.0468) (-23.9737, -23.8004) (-24.0265, -23.5805) knots 0 0 0 1 2 2 2
  line L108 (-24.0265, -23.5805) -> (-22.2552, -23.5805)
  spline S57 degree 2 poles (-22.2552, -23.5805) (-22.2493, -23.5365) (-22.2405, -23.4368) (-22.2405, -23.3987) knots 0 0 0 1 2 2 2
  spline S58 degree 2 poles (-23.4546, -22.6948) (-23.2229, -22.6977) (-22.9209, -22.9588) (-22.8798, -23.1846) knots 0 0 0 1 2 2 2
  line L109 (-22.8798, -23.1846) -> (-24.0353, -23.1846)
  spline S59 degree 2 poles (-24.0353, -23.1846) (-23.9972, -22.9558) (-23.6892, -22.6977) (-23.4546, -22.6948) knots 0 0 0 1 2 2 2
  spline S60 degree 2 poles (-0.9243, -24.6128) (-0.4902, -24.6099) (0.0846, -24.3518) (0.3691, -23.9265) (0.3691, -23.6685) knots 0 0 0 1 2 3 3 3
  spline S61 degree 2 poles (0.3691, -23.6685) (0.3632, -23.3371) (0.0083, -22.9763) (-0.5195, -22.8033) (-1.0445, -22.6948) (-1.3994, -22.5364) (-1.4052, -22.3722) knots 0 0 0 1 2 3 4 5 5 5
  spline S62 degree 2 poles (-1.4052, -22.3722) (-1.4081, -22.2256) (-1.1354, -22.0262) (-0.8245, -22.0232) knots 0 0 0 1 2 2 2
  spline S63 degree 2 poles (-0.8245, -22.0232) (-0.6222, -22.0232) (-0.1911, -22.1435) (0.0201, -22.2637) knots 0 0 0 1 2 2 2
  line L110 (0.0201, -22.2637) -> (0.2371, -21.727)
  spline S64 degree 2 poles (0.2371, -21.727) (0.023, -21.5921) (-0.5283, -21.4572) (-0.8216, -21.4572) knots 0 0 0 1 2 2 2
  spline S65 degree 2 poles (-0.8216, -21.4572) (-1.2527, -21.4601) (-1.8246, -21.7153) (-2.1061, -22.1435) (-2.1061, -22.4074) knots 0 0 0 1 2 3 3 3
  spline S66 degree 2 poles (-2.1061, -22.4074) (-2.1003, -22.7417) (-1.7454, -23.1054) (-1.2175, -23.2843) (-0.6926, -23.3928) (-0.3377, -23.5541) (-0.3319, -23.7213) knots 0 0 0 1 2 3 4 5 5 5
  spline S67 degree 2 poles (-0.3319, -23.7213) (-0.3289, -23.862) (-0.6105, -24.0438) (-0.9213, -24.0468) knots 0 0 0 1 2 2 2
  spline S68 degree 2 poles (-0.9213, -24.0468) (-1.1999, -24.0438) (-1.7307, -23.8708) (-1.9272, -23.73) knots 0 0 0 1 2 2 2
  line L111 (-1.9272, -23.73) -> (-2.1677, -24.2609)
  spline S69 degree 2 poles (-2.1677, -24.2609) (-1.9566, -24.4192) (-1.2967, -24.6099) (-0.9243, -24.6128) knots 0 0 0 1 2 2 2
  line L112 (3.9645, -22.2168) -> (3.3927, -23.8034)
  line L113 (3.3927, -23.8034) -> (2.8355, -22.2168)
  line L114 (2.8355, -22.2168) -> (2.2606, -22.2168)
  line L115 (2.2606, -22.2168) -> (1.6858, -23.8034)
  line L116 (1.6858, -23.8034) -> (1.1316, -22.2168)
  line L117 (1.1316, -22.2168) -> (0.4922, -22.2168)
  line L118 (0.4922, -22.2168) -> (1.3369, -24.56)
  line L119 (1.3369, -24.56) -> (1.9908, -24.56)
  line L120 (1.9908, -24.56) -> (2.5363, -23.1054)
  line L121 (2.5363, -23.1054) -> (3.0613, -24.56)
  line L122 (3.0613, -24.56) -> (3.7153, -24.56)
  line L123 (3.7153, -24.56) -> (4.5657, -22.2168)
  line L124 (4.5657, -22.2168) -> (3.9645, -22.2168)
  line L125 (4.8825, -24.56) -> (5.5629, -24.56)
  line L126 (5.5629, -24.56) -> (5.5629, -22.2168)
  line L127 (5.5629, -22.2168) -> (4.8825, -22.2168)
  line L128 (4.8825, -22.2168) -> (4.8825, -24.56)
  spline S70 degree 2 poles (5.2227, -21.8883) (5.4133, -21.8854) (5.642, -21.6684) (5.645, -21.4983) knots 0 0 0 1 2 2 2
  spline S71 degree 2 poles (5.645, -21.4983) (5.642, -21.337) (5.4133, -21.1346) (5.2227, -21.1317) knots 0 0 0 1 2 2 2
  spline S72 degree 2 poles (5.2227, -21.1317) (5.032, -21.1346) (4.8033, -21.3458) (4.8004, -21.51) knots 0 0 0 1 2 2 2
  spline S73 degree 2 poles (4.8004, -21.51) (4.8033, -21.6742) (5.032, -21.8854) (5.2227, -21.8883) knots 0 0 0 1 2 2 2
  spline S74 degree 2 poles (7.5219, -23.9676) (7.4662, -24.0116) (7.3225, -24.0556) (7.2462, -24.0556) knots 0 0 0 1 2 2 2
  spline S75 degree 2 poles (7.2462, -24.0556) (7.1084, -24.0556) (6.9559, -23.8972) (6.9559, -23.7476) knots 0 0 0 1 2 2 2
  line L129 (6.9559, -23.7476) -> (6.9559, -22.7916)
  line L130 (6.9559, -22.7916) -> (7.5395, -22.7916)
  line L131 (7.5395, -22.7916) -> (7.5395, -22.2696)
  line L132 (7.5395, -22.2696) -> (6.9559, -22.2696)
  line L133 (6.9559, -22.2696) -> (6.9559, -21.7006)
  line L134 (6.9559, -21.7006) -> (6.2755, -21.7006)
  line L135 (6.2755, -21.7006) -> (6.2755, -22.2696)
  line L136 (6.2755, -22.2696) -> (5.9148, -22.2696)
  line L137 (5.9148, -22.2696) -> (5.9148, -22.7916)
  line L138 (5.9148, -22.7916) -> (6.2755, -22.7916)
  line L139 (6.2755, -22.7916) -> (6.2755, -23.7535)
  spline S76 degree 2 poles (6.2755, -23.7535) (6.2784, -24.1729) (6.733, -24.5952) (7.1524, -24.5952) knots 0 0 0 1 2 2 2
  spline S77 degree 2 poles (7.1524, -24.5952) (7.3107, -24.5952) (7.5981, -24.5219) (7.7037, -24.4486) knots 0 0 0 1 2 2 2
  line L140 (7.7037, -24.4486) -> (7.5219, -23.9676)
  spline S78 degree 2 poles (9.2199, -24.5952) (9.5924, -24.5923) (10.1379, -24.2873) (10.2698, -24.0028) knots 0 0 0 1 2 2 2
  line L141 (10.2698, -24.0028) -> (9.7419, -23.7154)
  spline S79 degree 2 poles (9.7419, -23.7154) (9.6452, -23.8855) (9.3754, -24.038) (9.2141, -24.038) knots 0 0 0 1 2 2 2
  spline S80 degree 2 poles (9.2141, -24.038) (8.9501, -24.035) (8.607, -23.6978) (8.6011, -23.3869) knots 0 0 0 1 2 2 2
  spline S81 degree 2 poles (8.6011, -23.3869) (8.607, -23.079) (8.9501, -22.7417) (9.2141, -22.7388) knots 0 0 0 1 2 2 2
  spline S82 degree 2 poles (9.2141, -22.7388) (9.3754, -22.7388) (9.6452, -22.8942) (9.7419, -23.0614) knots 0 0 0 1 2 2 2
  line L142 (9.7419, -23.0614) -> (10.2698, -22.7769)
  spline S83 degree 2 poles (10.2698, -22.7769) (10.1379, -22.4895) (9.5924, -22.1845) (9.2199, -22.1816) knots 0 0 0 1 2 2 2
  spline S84 degree 2 poles (9.2199, -22.1816) (8.8357, -22.1845) (8.2492, -22.4895) (7.9149, -23.0321) (7.9119, -23.3869) knots 0 0 0 1 2 3 3 3
  spline S85 degree 2 poles (7.9119, -23.3869) (7.9149, -23.7447) (8.2492, -24.2873) (8.8357, -24.5923) (9.2199, -24.5952) knots 0 0 0 1 2 3 3 3
  spline S86 degree 2 poles (12.0881, -22.1816) (11.8594, -22.1816) (11.481, -22.3224) (11.3432, -22.4602) knots 0 0 0 1 2 2 2
  line L143 (11.3432, -22.4602) -> (11.3432, -21.3282)
  line L144 (11.3432, -21.3282) -> (10.6628, -21.3282)
  line L145 (10.6628, -21.3282) -> (10.6628, -24.56)
  line L146 (10.6628, -24.56) -> (11.3432, -24.56)
  line L147 (11.3432, -24.56) -> (11.3432, -23.3987)
  spline S87 degree 2 poles (11.3432, -23.3987) (11.3461, -23.0761) (11.6541, -22.7681) (11.9033, -22.7681) knots 0 0 0 1 2 2 2
  spline S88 degree 2 poles (11.9033, -22.7681) (12.1321, -22.7681) (12.3784, -23.0379) (12.3784, -23.3224) knots 0 0 0 1 2 2 2
  line L148 (12.3784, -23.3224) -> (12.3784, -24.56)
  line L149 (12.3784, -24.56) -> (13.0588, -24.56)
  line L150 (13.0588, -24.56) -> (13.0588, -23.2168)
  spline S89 degree 2 poles (13.0588, -23.2168) (13.0559, -22.862) (12.8037, -22.4015) (12.3667, -22.1816) (12.0881, -22.1816) knots 0 0 0 1 2 3 3 3
  line L151 (40.0181, -21.51) -> (39.0767, -23.689)
  line L152 (39.0767, -23.689) -> (38.15, -21.51)
  line L153 (38.15, -21.51) -> (37.3875, -21.51)
  line L154 (37.3875, -21.51) -> (38.7013, -24.56)
  line L155 (38.7013, -24.56) -> (39.3993, -24.56)
  line L156 (39.3993, -24.56) -> (40.719, -21.51)
  line L157 (40.719, -21.51) -> (40.0181, -21.51)
  spline S90 degree 2 poles (42.0182, -22.1816) (41.7337, -22.1816) (41.2058, -22.3282) (41.0093, -22.4631) knots 0 0 0 1 2 2 2
  line L158 (41.0093, -22.4631) -> (41.2527, -22.9412)
  spline S91 degree 2 poles (41.2527, -22.9412) (41.3818, -22.8385) (41.7396, -22.7212) (41.9273, -22.7212) knots 0 0 0 1 2 2 2
  spline S92 degree 2 poles (41.9273, -22.7212) (42.2, -22.7212) (42.4669, -22.9646) (42.4669, -23.1846) knots 0 0 0 1 2 2 2
  line L159 (42.4669, -23.1846) -> (41.9273, -23.1846)
  spline S93 degree 2 poles (41.9273, -23.1846) (41.3964, -23.1904) (40.9184, -23.5688) (40.9213, -23.8855) knots 0 0 0 1 2 2 2
  spline S94 degree 2 poles (40.9213, -23.8855) (40.9243, -24.1963) (41.3818, -24.5893) (41.7982, -24.5952) knots 0 0 0 1 2 2 2
  spline S95 degree 2 poles (41.7982, -24.5952) (42.0563, -24.5952) (42.417, -24.428) (42.5109, -24.2697) knots 0 0 0 1 2 2 2
  line L160 (42.5109, -24.2697) -> (42.5109, -24.56)
  line L161 (42.5109, -24.56) -> (43.1473, -24.56)
  line L162 (43.1473, -24.56) -> (43.1473, -23.2227)
  spline S96 degree 2 poles (43.1473, -23.2227) (43.1443, -22.6919) (42.5578, -22.1816) (42.0182, -22.1816) knots 0 0 0 1 2 2 2
  spline S97 degree 2 poles (41.9654, -24.1377) (41.7865, -24.1348) (41.5841, -23.9852) (41.5841, -23.8562) knots 0 0 0 1 2 2 2
  spline S98 degree 2 poles (41.5841, -23.8562) (41.5812, -23.7359) (41.766, -23.5834) (42.0006, -23.5805) knots 0 0 0 1 2 2 2
  line L163 (42.0006, -23.5805) -> (42.4669, -23.5805)
  line L164 (42.4669, -23.5805) -> (42.4669, -23.821)
  spline S99 degree 2 poles (42.4669, -23.821) (42.4053, -23.9793) (42.1384, -24.1377) (41.9654, -24.1377) knots 0 0 0 1 2 2 2
  line L165 (43.7602, -24.56) -> (44.4406, -24.56)
  line L166 (44.4406, -24.56) -> (44.4406, -21.3282)
  line L167 (44.4406, -21.3282) -> (43.7602, -21.3282)
  line L168 (43.7602, -21.3282) -> (43.7602, -24.56)
  line L169 (46.7427, -22.2168) -> (46.0712, -23.8122)
  line L170 (46.0712, -23.8122) -> (45.423, -22.2168)
  line L171 (45.423, -22.2168) -> (44.7221, -22.2168)
  line L172 (44.7221, -22.2168) -> (45.7075, -24.56)
  line L173 (45.7075, -24.56) -> (46.4084, -24.56)
  line L174 (46.4084, -24.56) -> (47.3967, -22.2168)
  line L175 (47.3967, -22.2168) -> (46.7427, -22.2168)
  spline S100 degree 2 poles (50.042, -23.3987) (50.0391, -23.0174) (49.7194, -22.4749) (49.171, -22.1845) (48.822, -22.1816) knots 0 0 0 1 2 3 3 3
  spline S101 degree 2 poles (48.822, -22.1816) (48.4613, -22.1845) (47.9012, -22.4925) (47.5756, -23.035) (47.5727, -23.3899) knots 0 0 0 1 2 3 3 3
  spline S102 degree 2 poles (47.5727, -23.3899) (47.5756, -23.7388) (47.9041, -24.2814) (48.5024, -24.5923) (48.91, -24.5952) knots 0 0 0 1 2 3 3 3
  spline S103 degree 2 poles (48.91, -24.5952) (49.2267, -24.5952) (49.7136, -24.4016) (49.8778, -24.2169) knots 0 0 0 1 2 2 2
  line L176 (49.8778, -24.2169) -> (49.5141, -23.8239)
  spline S104 degree 2 poles (49.5141, -23.8239) (49.3968, -23.9383) (49.1124, -24.0497) (48.9276, -24.0497) knots 0 0 0 1 2 2 2
  spline S105 degree 2 poles (48.9276, -24.0497) (48.6578, -24.0468) (48.3088, -23.8004) (48.256, -23.5805) knots 0 0 0 1 2 2 2
  line L177 (48.256, -23.5805) -> (50.0274, -23.5805)
  spline S106 degree 2 poles (50.0274, -23.5805) (50.0332, -23.5365) (50.042, -23.4368) (50.042, -23.3987) knots 0 0 0 1 2 2 2
  spline S107 degree 2 poles (48.8279, -22.6948) (49.0596, -22.6977) (49.3616, -22.9588) (49.4027, -23.1846) knots 0 0 0 1 2 2 2
  line L178 (49.4027, -23.1846) -> (48.2472, -23.1846)
  spline S108 degree 2 poles (48.2472, -23.1846) (48.2853, -22.9558) (48.5933, -22.6977) (48.8279, -22.6948) knots 0 0 0 1 2 2 2
  line L179 (67.1503, -24.56) -> (68.5346, -24.56)
  spline S109 degree 2 poles (68.5346, -24.56) (69.039, -24.5571) (69.7927, -24.1817) (70.215, -23.4984) (70.2179, -23.035) knots 0 0 0 1 2 3 3 3
  spline S110 degree 2 poles (70.2179, -23.035) (70.215, -22.5716) (69.7927, -21.8883) (69.039, -21.5129) (68.5346, -21.51) knots 0 0 0 1 2 3 3 3
  line L180 (68.5346, -21.51) -> (67.1503, -21.51)
  line L181 (67.1503, -21.51) -> (67.1503, -24.56)
  line L182 (67.8571, -23.9793) -> (67.8571, -22.0907)
  line L183 (67.8571, -22.0907) -> (68.5023, -22.0907)
  spline S111 degree 2 poles (68.5023, -22.0907) (68.9598, -22.0936) (69.4965, -22.5922) (69.5024, -23.035) knots 0 0 0 1 2 2 2
  spline S112 degree 2 poles (69.5024, -23.035) (69.4965, -23.4778) (68.9598, -23.9764) (68.5023, -23.9793) knots 0 0 0 1 2 2 2
  line L184 (68.5023, -23.9793) -> (67.8571, -23.9793)
  line L185 (71.35, -22.5247) -> (71.35, -22.2168)
  line L186 (71.35, -22.2168) -> (70.7018, -22.2168)
  line L187 (70.7018, -22.2168) -> (70.7018, -24.56)
  line L188 (70.7018, -24.56) -> (71.3822, -24.56)
  line L189 (71.3822, -24.56) -> (71.3822, -23.4544)
  spline S113 degree 2 poles (71.3822, -23.4544) (71.3852, -23.1171) (71.7195, -22.8004) (72.004, -22.8004) knots 0 0 0 1 2 2 2
  spline S114 degree 2 poles (72.004, -22.8004) (72.0421, -22.8004) (72.1154, -22.8063) (72.1565, -22.8092) knots 0 0 0 1 2 2 2
  line L190 (72.1565, -22.8092) -> (72.1565, -22.1816)
  spline S115 degree 2 poles (72.1565, -22.1816) (71.8837, -22.1816) (71.4761, -22.3546) (71.35, -22.5247) knots 0 0 0 1 2 2 2
  line L191 (74.2504, -22.2168) -> (73.5876, -23.8063)
  line L192 (73.5876, -23.8063) -> (72.9307, -22.2168)
  line L193 (72.9307, -22.2168) -> (72.2298, -22.2168)
  line L194 (72.2298, -22.2168) -> (73.2445, -24.5776)
  line L195 (73.2445, -24.5776) -> (73.2357, -24.6011)
  spline S116 degree 2 poles (73.2357, -24.6011) (73.1682, -24.7565) (72.9923, -24.8943) (72.8515, -24.8914) knots 0 0 0 1 2 2 2
  spline S117 degree 2 poles (72.8515, -24.8914) (72.7489, -24.8914) (72.5494, -24.8122) (72.4702, -24.7448) knots 0 0 0 1 2 2 2
  line L196 (72.4702, -24.7448) -> (72.221, -25.2257)
  spline S118 degree 2 poles (72.221, -25.2257) (72.3383, -25.3284) (72.6902, -25.4398) (72.875, -25.4398) knots 0 0 0 1 2 2 2
  spline S119 degree 2 poles (72.875, -25.4398) (73.1917, -25.4457) (73.6756, -25.1201) (73.8457, -24.7037) knots 0 0 0 1 2 2 2
  line L197 (73.8457, -24.7037) -> (74.9044, -22.2168)
  line L198 (74.9044, -22.2168) -> (74.2504, -22.2168)
  spline S120 degree 2 poles (-59.4673, -9.7858) (-58.8134, -9.782) (-57.798, -9.2435) (-57.2211, -8.3051) (-57.2134, -7.6935) knots 0 0 0 1 2 3 3 3
  spline S121 degree 2 poles (-57.2134, -7.6935) (-57.2211, -7.082) (-57.798, -6.1435) (-58.8134, -5.6051) (-59.4673, -5.6012) knots 0 0 0 1 2 3 3 3
  spline S122 degree 2 poles (-59.4673, -5.6012) (-60.125, -5.6051) (-61.1404, -6.1435) (-61.7173, -7.082) (-61.725, -7.6935) knots 0 0 0 1 2 3 3 3
  spline S123 degree 2 poles (-61.725, -7.6935) (-61.7173, -8.3051) (-61.1404, -9.2435) (-60.125, -9.782) (-59.4673, -9.7858) knots 0 0 0 1 2 3 3 3
  spline S124 degree 2 poles (-59.4673, -8.6935) (-59.8519, -8.6897) (-60.3596, -8.1666) (-60.3673, -7.6935) knots 0 0 0 1 2 2 2
  spline S125 degree 2 poles (-60.3673, -7.6935) (-60.3596, -7.2204) (-59.8519, -6.6974) (-59.4673, -6.6935) knots 0 0 0 1 2 2 2
  spline S126 degree 2 poles (-59.4673, -6.6935) (-59.0865, -6.6974) (-58.5788, -7.2204) (-58.5711, -7.6935) knots 0 0 0 1 2 2 2
  spline S127 degree 2 poles (-58.5711, -7.6935) (-58.5788, -8.1666) (-59.0865, -8.6897) (-59.4673, -8.6935) knots 0 0 0 1 2 2 2
  spline S128 degree 2 poles (-55.5404, -9.7512) (-54.998, -9.7474) (-54.2827, -9.4589) (-53.925, -8.982) (-53.925, -8.6935) knots 0 0 0 1 2 3 3 3
  spline S129 degree 2 poles (-53.925, -8.6935) (-53.9327, -8.3243) (-54.2904, -7.9281) (-54.8211, -7.7551) (-55.3519, -7.6974) (-55.7096, -7.632) (-55.7173, -7.5397) knots 0 0 0 1 2 3 4 5 5 5
  spline S130 degree 2 poles (-55.7173, -7.5397) (-55.7211, -7.482) (-55.5404, -7.3935) (-55.2942, -7.3935) knots 0 0 0 1 2 2 2
  spline S131 degree 2 poles (-55.2942, -7.3935) (-55.098, -7.3897) (-54.6365, -7.4897) (-54.3942, -7.6204) knots 0 0 0 1 2 2 2
  line L199 (-54.3942, -7.6204) -> (-54.0404, -6.7704)
  spline S132 degree 2 poles (-54.0404, -6.7704) (-54.2942, -6.6435) (-54.9634, -6.5127) (-55.3134, -6.5127) knots 0 0 0 1 2 2 2
  spline S133 degree 2 poles (-55.3134, -6.5127) (-55.8365, -6.5166) (-56.548, -6.8012) (-56.9096, -7.282) (-56.9096, -7.582) knots 0 0 0 1 2 3 3 3
  spline S134 degree 2 poles (-56.9096, -7.582) (-56.9019, -7.9512) (-56.5442, -8.3474) (-56.0096, -8.5127) (-55.4788, -8.5704) (-55.1211, -8.632) (-55.1134, -8.7204) knots 0 0 0 1 2 3 4 5 5 5
  spline S135 degree 2 poles (-55.1134, -8.7204) (-55.1096, -8.7897) (-55.2827, -8.8704) (-55.5134, -8.8704) knots 0 0 0 1 2 2 2
  spline S136 degree 2 poles (-55.5134, -8.8704) (-55.7942, -8.8704) (-56.375, -8.7243) (-56.6019, -8.5897) knots 0 0 0 1 2 2 2
  line L200 (-56.6019, -8.5897) -> (-56.9557, -9.4435)
  spline S137 degree 2 poles (-56.9557, -9.4435) (-56.7057, -9.582) (-55.9519, -9.7474) (-55.5404, -9.7512) knots 0 0 0 1 2 2 2
  spline S138 degree 2 poles (-49.4019, -6.5127) (-49.725, -6.5127) (-50.2557, -6.7589) (-50.4442, -6.9858) knots 0 0 0 1 2 2 2
  spline S139 degree 2 poles (-50.4442, -6.9858) (-50.6096, -6.7435) (-51.1134, -6.5127) (-51.4211, -6.5127) knots 0 0 0 1 2 2 2
  spline S140 degree 2 poles (-51.4211, -6.5127) (-51.6788, -6.5127) (-52.1288, -6.6858) (-52.3057, -6.8627) knots 0 0 0 1 2 2 2
  line L201 (-52.3057, -6.8627) -> (-52.3057, -6.5704)
  line L202 (-52.3057, -6.5704) -> (-53.5365, -6.5704)
  line L203 (-53.5365, -6.5704) -> (-53.5365, -9.6935)
  line L204 (-53.5365, -9.6935) -> (-52.2442, -9.6935)
  line L205 (-52.2442, -9.6935) -> (-52.2442, -8.1666)